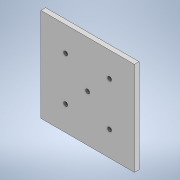
# Autodesk Inventor part: AlignmentPlate
Saved by Autodesk Inventor 2021 (Build 250183000, 183)
## iProperties
Created: 2020-03-15
Part Number: AlignmentPlate
Material: Generic
Document SubType Name: Modeling
Designer: elmar
Density: 1 g/cm^3
Appearance: Default
Author: elmar
Autodesk Inventor part; units mm, degrees
ref_plane "YZ Plane" through (0, 0, 0) normal (1, 0, 0) x (0, 1, 0)
ref_plane "XZ Plane" through (0, 0, 0) normal (0, 1, 0) x (-1, 0, 0)
ref_plane "XY Plane" through (0, 0, 0) normal (0, 0, 1) x (1, 0, 0)
sketch "Sketch41" plane through (0, 0, 0) normal (0, 0, 1) x (1, 0, 0)
  line L0 (80, -80) -> (-80, -80)
  line L1 (-80, -80) -> (-80, 80)
  line L2 (-80, 80) -> (80, 80)
  line L3 (80, 80) -> (80, -80)
  line L4 (80, -80) -> (-80, 80) construction
  line L5 (-80, -80) -> (80, 80) construction
  circle A0 centre (-37.5, 37.5) radius 37.5
  line L6 (0, -112) -> (0, 112) projected
  line L7 (-112, 0) -> (112, 0) projected
  circle A1 centre (-37.5, 37.5) radius 31.6165
  circle A2 centre (-37.5, 37.5) radius 21.4165
  circle A3 centre (37.5, -37.5) radius 31.6165
  circle A4 centre (37.5, -37.5) radius 21.4165
  line L8 (59.8562, -15.1438) -> (-15.1438, 59.8562)
  line L9 (52.6438, -22.3562) -> (-22.3562, 52.6438)
  line L10 (15.1438, -59.8562) -> (-59.8562, 15.1438)
  line L11 (22.3562, -52.6438) -> (-52.6438, 22.3562)
  circle A5 centre (-37.5, -37.5) radius 31.6165
  circle A6 centre (-37.5, -37.5) radius 21.4165
  circle A7 centre (37.5, 37.5) radius 31.6165
  circle A8 centre (37.5, 37.5) radius 21.4165
  line L12 (59.8562, 15.1438) -> (-15.1438, -59.8562)
  line L13 (52.6438, 22.3562) -> (-22.3562, -52.6438)
  line L14 (15.1438, 59.8562) -> (-59.8562, -15.1438)
  line L15 (22.3562, 52.6438) -> (-52.6438, -22.3562)
  line L16 (-37.5, 37.5) -> (-37.5, -37.5)
  circle A9 centre (-60.481, 60.481) radius 5
  line L17 (-49.8744, 49.8744) -> (-71.0876, 71.0876)
  arc A10 (-49.8744, 49.8744) -> (-71.0876, 71.0876) centre (-74.6231, 46.3388) ccw
  arc A11 (-71.0876, 71.0876) -> (-49.8744, 49.8744) centre (-46.3388, 74.6231) ccw
  arc A12 (-49.6403, 49.6403) -> (-71.3216, 71.3216) centre (-74.6231, 46.3388) ccw
  arc A13 (-71.3216, 71.3216) -> (-49.6403, 49.6403) centre (-46.3388, 74.6231) ccw
  line L18 (53.6853, -18.7098) -> (35.2271, 4.9396)
  circle A14 centre (44.4562, -6.8851) radius 5
  arc A15 (35.2271, 4.9396) -> (53.6853, -18.7098) centre (60.2225, 5.4203) ccw
  arc A16 (53.6853, -18.7098) -> (35.2271, 4.9396) centre (28.6899, -19.1906) ccw
  circle A17 centre (-37.5, 37.5) radius 17.5
  circle A18 centre (-37.5, 37.5) radius 7.5
  line L19 (-71.3216, 71.3216) -> (-49.6403, 49.6403)
  line L20 (-52.6438, 22.3562) -> (-59.8562, 15.1438)
  arc A19 (-62.7512, 26.1128) -> (-44.7125, 0) centre (17.6641, 62.3766) ccw
  arc A20 (-53.4529, 30.3059) -> (-37.5, 7.2125) centre (17.6641, 62.3766) ccw
  arc A21 (0, 44.7125) -> (-26.1128, 62.7512) centre (-62.3766, -17.6641) ccw
  arc A22 (-7.2125, 37.5) -> (-30.3059, 53.4529) centre (-62.3766, -17.6641) ccw
  line L21 (-37.5, 37.5) -> (-26.1128, 62.7512)
  circle A23 centre (-37.5, 37.5) radius 27.7
  circle A24 centre (-65.9013, 65.9013) radius 7.6655
  line L22 (-73.1417, 68.4185) -> (-44.18, 58.3498)
  line L23 (-73.5645, 66.0883) -> (-42.9116, 65.3403)
  line L24 (-73.038, 68.6991) -> (-44.4913, 57.5078)
  line L25 (-30.2936, 64.2462) -> (-63.9071, 73.3029)
  line L26 (-32.9472, 54.3974) -> (-44.4913, 57.5078)
  arc A25 (-60.0448, 43.663) -> (-44.4913, 57.5078) centre (-65.9013, 65.9013) ccw
  line L27 (-64.2462, 30.2936) -> (-73.3029, 63.9071)
  line L28 (-54.3974, 32.9472) -> (-57.5078, 44.4913)
  point P0 (0, 0)
  point P1 (-37.5, 7.2125)
  point P2 (44.7125, 0)
  point P3 (-30.2875, 0)
  point P4 (-60.481, 60.481)
  dimension "d1039" = 35
  dimension "TrackWidth" = 10.2
  dimension "d715" = 160
  dimension "d718" = 75
  dimension "d721" = 10
  dimension "d722" = 30
  dimension "d723" = 0.2
  dimension "d1003" = 10
  dimension "d1004" = 30
  dimension "d1040" = 15
  constraints: 54 end point, 32 point on circle, 17 centre point, 17 point on line, 15 symmetric about line, 11 tangent, 8 coincident, 5 horizontal, 4 equal length, 4 midpoint, 4 parallel, 3 perpendicular, 2 equal radius, 1 concentric, 61 other
  measures "d715" distance of L1.end L2.end
  measures "d718" diameter of A0
  measures "d721" diameter of A9
  measures "d722" distance of L17.end L17.start
  measures "d723" radial gap between concentric circles of A10 A12
  measures "d1003" diameter of A14
  measures "d1004" distance of L18.start L18.end
  measures "d1040" diameter of A18
extrude "Extrusion39" add sketch "Sketch41" along normal blind 8
hole "Hole11" at (37.5, 37.5, 0) at (-37.5, 37.5, 0) at (-37.5, -37.5, 0) at (0, 0, 0) at (37.5, -37.5, 0) direction (0, 0, 1) diameter 7 end through all countersink diameter 8 countersink angle 8
equation "\"TrackClearance\" = 0.2"
equation "\"d903\" = 55deg"
equation "\"Sketch59_Pitch\" = 1.25"
equation "\"d921\" = 55deg"
equation "\"Sketch61_Pitch\" = 1.25"
equation "\"d939\" = 55deg"
equation "\"Sketch63_Pitch\" = 1.25"
equation "\"d957\" = 55deg"
equation "\"Sketch65_Pitch\" = 1.25"
equation "\"d975\" = 55deg"
equation "\"Sketch67_Pitch\" = 1.25"
equation "\"d1117\" = 55deg"
equation "\"Sketch85_Pitch\" = 1.25"
equation "\"d1140\" = 55deg"
equation "\"Sketch87_Pitch\" = 1.25"
equation "\"d1160\" = 55deg"
equation "\"Sketch89_Pitch\" = 1.25"
equation "\"d1180\" = 55deg"
equation "\"Sketch91_Pitch\" = 1.25"
equation "\"d1202\" = 55deg"
equation "\"Sketch94_Pitch\" = 1.25"
